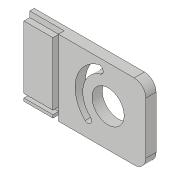
# Autodesk Inventor part: Lidar Sensor Case v4 Piece 2
Saved by Autodesk Inventor 2018.3 (Build 223284000, 284)
## iProperties
Created: 2019-03-27
Part Number: Lidar Sensor Case v4 Piece 2
Material: Generic
Document SubType Name: Modeling
Designer: aye06091
Mass: 12.4743 g
Surface Area: 69.2649 cm^2
Volume: 12.4743 cm^3
Density: 1 g/cm^3
Appearance: Default
Author: aye06091
Autodesk Inventor part; units mm, degrees
ref_plane "YZ Plane" through (0, 0, 0) normal (1, 0, 0) x (0, 1, 0)
ref_plane "XZ Plane" through (0, 0, 0) normal (0, 1, 0) x (-1, 0, 0)
ref_plane "XY Plane" through (0, 0, 0) normal (0, 0, 1) x (1, 0, 0)
sketch "Sketch1" plane through (0, 0, 0) normal (0, 0, 1) x (1, 0, 0)
  line L0 (0, 0) -> (66.675, 0)
  line L1 (66.675, 0) -> (66.675, -41.275)
  line L2 (66.675, -41.275) -> (0, -41.275)
  line L3 (0, -41.275) -> (0, 0)
  arc A0 (40.6531, -3.4261) -> (33.474, -33.5752) centre (46.0375, -20.6375) ccw
  arc A1 (41.8969, -7.4017) -> (36.376, -30.5868) centre (46.0375, -20.6375) ccw
  arc A2 (41.8969, -7.4017) -> (40.6531, -3.4261) centre (41.275, -5.4139) ccw
  arc A3 (33.474, -33.5752) -> (36.376, -30.5868) centre (34.925, -32.081) ccw
  circle A4 centre (46.0375, -20.6375) radius 8.7948
  dimension "d0" = 41.275
  dimension "d1" = 66.675
  dimension "d8" = 17.5895
  dimension "d9" = 20.6375
  dimension "d25" = 20.6375
  dimension "d32" = 25.4
  dimension "d33" = 31.75
  dimension "d49" = 2.0828
  dimension "d50" = 15.9512
  constraints: 8 end point, 8 point on circle, 5 centre point, 4 tangent, 2 coincident, 2 parallel, 1 horizontal, 1 perpendicular
  measures "d0" distance of L2.end L0.start
  measures "d1" distance of L0.start L0.end
  measures "d8" diameter of A4
  measures "d9" distance from line of L0 A0.centre
  measures "d25" distance from line of L1 A0.centre
  measures "d32" distance from line of L1 A2.centre
  measures "d33" distance from line of L1 A3.centre
  measures "d49" radius of A2
  measures "d50" distance of A0.centre A2.centre
extrude "Extrusion1" add sketch "Sketch1" against normal blind 5.6134
sketch "Sketch3" plane through (0, 0, 0) normal (0, 0, 1) x (1, 0, 0)
  line L0 (0, 0) -> (66.675, 0) projected
  line L1 (0, -41.275) -> (0, 0) projected
  line L2 (66.675, -41.275) -> (0, -41.275) projected
  line L3 (0, 0) -> (18.8976, 0)
  line L4 (18.8976, 0) -> (18.8976, -3.175)
  line L5 (18.8976, -3.175) -> (0, -3.175)
  line L6 (0, -3.175) -> (0, 0)
  line L7 (18.8976, 0) -> (15.875, 0)
  line L8 (15.875, 0) -> (15.875, -41.275)
  line L9 (15.875, -41.275) -> (18.8976, -41.275)
  line L10 (18.8976, -41.275) -> (18.8976, 0)
  line L11 (15.875, -41.275) -> (15.875, -3.175)
  line L12 (15.875, -41.275) -> (0, -41.275)
  line L13 (0, -41.275) -> (0, 0)
  line L14 (0, -39.6875) -> (15.875, -39.6875)
  line L15 (15.875, -39.6875) -> (15.875, -37.5285)
  line L16 (15.875, -37.5285) -> (0, -37.5285)
  line L17 (0, -37.5285) -> (0, -39.6875)
  dimension "d26" = 15.875
  dimension "d27" = 3.0226
  dimension "d28" = 3.175
  dimension "d38" = 1.5875
  dimension "d39" = 2.159
  constraints: 30 end point, 6 parallel, 3 horizontal, 3 perpendicular, 3 point on line
  measures "d26" distance between parallel lines of L1 L8
  measures "d27" distance between parallel lines of L10 L8
  measures "d28" distance between parallel lines of L0 L5
  measures "d38" distance between parallel lines of L12 L14
  measures "d39" distance between parallel lines of L16 L14
extrude "Extrusion3" cut sketch "Sketch3" against normal blind 3.175 contours L0 L8 L5 L1 | L0 L4 L5 L8 | L5 L10 L2 L8 | L16 L8 L14 L1
fillet "Fillet1" radius 6.35 2 edges at (66.675, 0, -2.8067) (66.675, -41.275, -2.8067)
body "Solid1"
